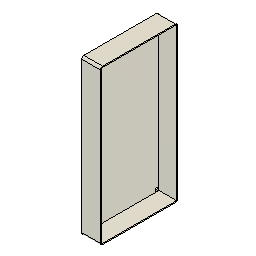
Back Door (Autodesk Fusion 360 design; units mm, degrees)
Autodesk Fusion 360 part; units mm, degrees
note: some values were not read from the file. Set by a fixed rule: which sketch regions a step uses.
sketch "Sketch1" plane through (0, 0, 0) normal (1, 0, 0) x (0, 0, -1)
  line L0 (35, -70) -> (-35, -70)
  line L1 (-35, -70) -> (-35, 70)
  line L2 (-35, 70) -> (35, 70)
  line L3 (35, 70) -> (35, -70)
  line L4 (35, -70) -> (-35, 70) construction
  line L5 (-35, -70) -> (35, 70) construction
  dimension "d1" = 70
  dimension "d2" = 140
  constraint horizontal L0
  constraint perpendicular L0 L1
  constraint parallel L0 L2
  constraint parallel L1 L3
  constraint coincident L4 origin
  constraint coincident L5 origin
  measures "d1" distance of L1.end L2.end
  measures "d2" distance of L0.end L1.end
extrude "Extrude1" add sketch "Sketch1" along normal blind 17
shell "Shell1" thickness 1 removed faces 1 at (17, -23.3333, 11.6667)
fillet "Fillet1" radius 2 1 edges at (8.5, 70, 35)
fillet "Fillet1" radius 2 1 edges at (8.5, 70, -35)
fillet "Fillet1" radius 2 1 edges at (8.5, -70, 35)
fillet "Fillet1" radius 2 1 edges at (8.5, -70, -35)
sketch "Sketch2" plane through (0, 0, 0) normal (-1, 0, 0) x (0, 0, 1)
  arc A0 (-35, -68) -> (-33, -70) centre (-33, -68) ccw
  line L0 (-33, -70) -> (33, -70)
  arc A1 (33, -70) -> (35, -68) centre (33, -68) ccw
  line L1 (35, -68) -> (35, 68)
  arc A2 (35, 68) -> (33, 70) centre (33, 68) ccw
  line L2 (33, 70) -> (-33, 70)
  arc A3 (-33, 70) -> (-35, 68) centre (-33, 68) ccw
  line L3 (-35, 68) -> (-35, -68)
  line L4 (32, 67) -> (-32, 67)
  line L5 (-32, 67) -> (-32, -67)
  line L6 (-32, -67) -> (32, -67)
  line L7 (32, -67) -> (32, 67)
  line L8 (32, 67) -> (-32, -67) construction
  line L9 (-32, 67) -> (32, -67) construction
  circle A4 centre (-32, 67) radius 1.5
  circle A5 centre (32, 67) radius 1.5
  circle A6 centre (32, -67) radius 1.5
  circle A7 centre (-32, -67) radius 1.5
  dimension "d14" = 64
  dimension "d15" = 134
  dimension "d16" = 3
  dimension "d17" = 3
  dimension "d18" = 3
  dimension "d19" = 3
  constraint horizontal L4
  constraint perpendicular L4 L5
  constraint parallel L4 L6
  constraint parallel L5 L7
  constraint coincident L8 origin
  constraint coincident L9 origin
  constraint coincident L4.end L5.start
  constraint coincident L4.start L7.end
  constraint coincident L6.end L7.start
  constraint coincident L5.end L6.start
  measures "d14" distance of L5.end L6.end
  measures "d15" distance of L4.end L5.end
  measures "d16" diameter of A4
  measures "d17" diameter of A5
  measures "d18" diameter of A6
  measures "d19" diameter of A7
extrude "Extrude2" cut sketch "Sketch2" against normal blind 10 contours L4 L5 A4 | L4 L5 A4 | L4 L7 A5 | L4 L7 A5 | L5 L6 A7 | L5 L6 A7 | L6 L7 A6 | L6 L7 A6
sketch "Sketch3" plane through (0, 0, 0) normal (-1, 0, 0) x (0, 0, 1)
  circle A0 centre (32, -67) radius 1.5
  circle A1 centre (32, 67) radius 1.5
  circle A2 centre (-32, -67) radius 1.5
  circle A3 centre (-32, 67) radius 1.5
  arc A4 (-35, -68) -> (-33, -70) centre (-33, -68) ccw
  line L0 (-33, -70) -> (33, -70)
  arc A5 (33, -70) -> (35, -68) centre (33, -68) ccw
  line L1 (35, -68) -> (35, 68)
  arc A6 (35, 68) -> (33, 70) centre (33, 68) ccw
  line L2 (33, 70) -> (-33, 70)
  arc A7 (-33, 70) -> (-35, 68) centre (-33, 68) ccw
  line L3 (-35, 68) -> (-35, -68)
  line L4 (0, 0) -> (10, 0)
  line L5 (10, 0) -> (-10, 0)
  line L6 (-10, 0) -> (-10, 35)
  line L7 (-10, 35) -> (-15, 35)
  line L8 (-15, 35) -> (-15, -35)
  line L9 (-15, -35) -> (-10, -35)
  line L10 (-10, -35) -> (-10, 0)
  line L11 (10, 0) -> (10, 35)
  line L12 (10, 35) -> (15, 35)
  line L13 (15, 35) -> (15, -35)
  line L14 (15, -35) -> (10, -35)
  line L15 (10, -35) -> (10, 0)
  constraint coincident L4.start origin
  constraint horizontal L4
  constraint parallel L4 L5
  constraint perpendicular L5 L6
  constraint perpendicular L6 L7
  constraint perpendicular L7 L8
  constraint perpendicular L6 L9
  constraint perpendicular L5 L10
  constraint perpendicular L7 L11
  constraint perpendicular L11 L12
  constraint perpendicular L9 L13
  constraint perpendicular L11 L14
  constraint perpendicular L4 L15
extrude "Extrude3" add sketch "Sketch3" along normal blind 3 contours L6 L7 L8 L9 L10 | L11 L12 L13 L14 L15
fillet "Fillet2" radius 1 1 edges at (-3, 0, 10)
fillet "Fillet2" radius 1 1 edges at (-3, 0, 15)
fillet "Fillet3" radius 1 1 edges at (-3, 0, -10)
fillet "Fillet4" radius 1 1 edges at (-3, 0, -15)
sketch "Sketch4" plane through (0, 35, 0) normal (0, 1, 0) x (-1, 0, 0)
  arc A0 (3, -11) -> (2, -10) centre (2, -11) ccw
  line L0 (2, -10) -> (0, -10)
  line L1 (0, -10) -> (0, -15)
  line L2 (0, -15) -> (2, -15)
  line L3 (0, -10) -> (2, -10)
  line L4 (2, -15) -> (0, -15)
  arc A1 (3, -11) -> (2, -10) centre (2, -11) ccw
  line L5 (0, -10) -> (0.5, -10)
  line L6 (0, -10) -> (0, -10.5)
  line L7 (1, -10.5) -> (0, -10.5)
  line L8 (0, -15) -> (0, -14.5)
  line L9 (0, -14.5) -> (1, -14.5)
  line L10 (0, -15) -> (0, -14.5)
  line L11 (0, -10.5) -> (0, -10)
  line L12 (1, -10) -> (1, -10.5)
  line L13 (1, -14.5) -> (1, -15)
  dimension "d32" = 1
  constraint horizontal L3
  constraint vertical L10
  constraint coincident L0.end L1.start
  constraint tangent L3 A1
  constraint coincident L3 L5.end
  constraint midpoint L0 L12.start
  constraint midpoint L2 L13.end
  constraint perpendicular L1 L7
  constraint coincident L1.end L2.start
  constraint coincident L1 L8.end
  constraint perpendicular L9 L13
  constraint collinear L10 L11
  constraint collinear L12 L13
  measures "d32" radius of A1
extrude "Extrude4" cut sketch "Sketch4" against normal blind 70
sketch "Sketch5" plane through (0, 35, 0) normal (0, 1, 0) x (-1, 0, 0)
  arc A0 (3, 14) -> (2, 15) centre (2, 14) ccw
  line L0 (2, 15) -> (0, 15)
  line L1 (0, 15) -> (0, 10)
  line L2 (0, 10) -> (2, 10)
  arc A1 (2, 10) -> (3, 11) centre (2, 11) ccw
  line L3 (3, 11) -> (3, 14)
  line L4 (0, 15) -> (1, 15)
  line L5 (1, 15) -> (1, 14.5)
  line L6 (1, 14.5) -> (0, 14.5)
  line L7 (0, 15) -> (0, 14.5)
  line L8 (0, 10) -> (0, 10.5)
  line L9 (1, 10.5) -> (1, 10)
  line L10 (0, 10.5) -> (1, 10.5)
  line L11 (1, 10) -> (0, 10)
  constraint coincident L0.end L1.start
  constraint midpoint L0 L4.end
  constraint perpendicular L0 L5
  constraint coincident L1 L6.end
  constraint perpendicular L1 L6
  constraint coincident L1.end L2.start
  constraint coincident L1 L8.end
  constraint midpoint L2 L9.end
  constraint perpendicular L2 L9
  constraint perpendicular L1 L10
extrude "Extrude5" cut sketch "Sketch5" against normal blind 70 contours L0 L1 L4 L5 L6 L7 | L1 L2 L8 L9 L10 L11
